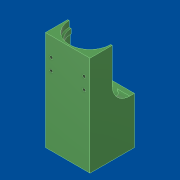
# Autodesk Inventor part: 402-gearbox-housing
Saved by Autodesk Inventor 2018 (Build 220112000, 112)
## iProperties
Created: 2020-06-11
Part Number: 402-gearbox-housing
Material: Generic
Document SubType Name: Modeling
Designer: Bunny320
Density: 1 g/cm^3
Appearance: Smooth - Dark Forest Green
Author: Bunny320
Autodesk Inventor part; units mm, degrees
ref_plane "YZ Plane" through (0, 0, 0) normal (1, 0, 0) x (0, 1, 0)
ref_plane "XZ Plane" through (0, 0, 0) normal (0, 1, 0) x (-1, 0, 0)
ref_plane "XY Plane" through (0, 0, 0) normal (0, 0, 1) x (1, 0, 0)
sketch "Sketch1" plane through (0, 0, 0) normal (0, 0, 1) x (1, 0, 0)
  line L0 (-19, -19) -> (19, -19)
  line L1 (19, -19) -> (19, 19)
  line L2 (19, 19) -> (-19, 19)
  line L3 (-19, 19) -> (-19, -19)
  line L4 (-19, -19) -> (19, 19) construction
  line L5 (19, -19) -> (-19, 19) construction
  point P0 (0, 0)
  dimension "d0" = 38
  constraints: 12 end point, 2 midpoint, 2 parallel, 2 perpendicular, 1 horizontal
  measures "d0" distance of L1.end L2.end
extrude "Extrusion1" add sketch "Sketch1" along normal blind 85
sketch "Sketch2" plane through (0, 0, 0) normal (0, 0, -1) x (-1, 0, 0)
  circle A0 centre (0, 0) radius 16.1
  dimension "d3" = 32.2
  constraints: 1 centre point, 1 coincident
  measures "d3" diameter of A0
extrude "Extrusion2" cut sketch "Sketch2" against normal blind 32
sketch "Sketch3" plane through (0, 0, 85) normal (0, 0, 1) x (1, 0, 0)
  circle A0 centre (0, 0) radius 17
  dimension "d6" = 34
  constraints: 1 centre point, 1 coincident
  measures "d6" diameter of A0
extrude "Extrusion3" cut sketch "Sketch3" against normal blind 45
sketch "Sketch4" plane through (0, 0, 40) normal (0, 0, 1) x (1, 0, 0)
  circle A0 centre (0, 0) radius 10
  dimension "d9" = 20
  constraints: 1 centre point, 1 coincident
  measures "d9" diameter of A0
extrude "Extrusion4" cut sketch "Sketch4" against normal through all
sketch "Sketch5" plane through (0, 0, 40) normal (0, 0, 1) x (1, 0, 0)
  point P0 (0, 0)
  point P1 (0, 13)
  dimension "d12" = 13
  constraints: 1 vertical alignment
  measures "d12" distance of point (0, 0) point (0, 13)
hole "Hole1" at (0, 13, 40) direction (0, 0, -1) diameter 3.4 end through all countersink diameter 7.5 countersink angle 90 clearance for "Countersunk Flat Head Hex Socket Screw DIN EN ISO 10642" size "M3" standard "DIN"
pattern_circular "Circular Pattern1" count 4 over 360 about axis through (0, 0, -10) along (0, 0, 1) of "Hole1"
sketch "Sketch7" plane through (0, 0, 0) normal (0, 1, 0) x (-1, 0, 0)
  line L0 (17, 55) -> (11, 55)
  line L1 (11, 55) -> (11, 63)
  line L2 (11, 63) -> (17, 63)
  line L3 (17, 85) -> (17, 40) projected
  line L4 (17, 63) -> (17, 55)
  line L5 (0, 87.7085) -> (0, 95.5721)
  line L6 (1.9638, 40) -> (9.8053, 40) projected
  line L7 (17, 77) -> (17, 64.9)
  line L8 (-17, 85) -> (17, 85) projected
  line L9 (17, 80) -> (16, 80)
  line L10 (16, 80) -> (16, 76)
  line L11 (16, 76) -> (17, 76)
  line L12 (17, 76) -> (17, 80)
  line L13 (17, 85) -> (17, 40) projected
  line L14 (-19, 0) -> (19, 0) projected
  line L15 (9.8053, 40) -> (16.75, 40) projected
  point P0 (0, 0)
  point P1 (0, 0)
  dimension "d27" = 22
  dimension "d39" = 5
  dimension "d40" = 9
  dimension "d41" = 32
  dimension "d90" = 8
  dimension "d92" = 15
  constraints: 21 end point, 4 perpendicular, 4 point on line, 2 collinear, 2 horizontal, 1 midpoint, 1 vertical
  measures "d27" diameter of L1 L5
  measures "d39" distance between parallel lines of L8 L9
  measures "d40" distance between parallel lines of L8 L11
  measures "d41" diameter of L10 L5
  measures "d90" distance between parallel lines of L2 L0
  measures "d92" distance between parallel lines of L15 L0
revolve "Revolution1" add sketch "Sketch7" angle 360 about axis through (0, 0, 87.7085) along (0, 0, 1)
sketch "Sketch8" plane through (0, 0, 85) normal (0, 0, 1) x (1, 0, 0)
  circle A0 centre (0, 0) radius 17.75
  dimension "d42" = 35.5
  constraints: 1 centre point, 1 coincident
  measures "d42" diameter of A0
extrude "Extrusion6" cut sketch "Sketch8" against normal up to surface (5 mm away)
sketch "Sketch10" plane through (-19, -19, 0) normal (0, -1, 0) x (1, 0, 0)
  line L0 (33, 70.95) -> (5, 70.95)
  line L1 (5, 70.95) -> (5, 65)
  line L2 (5, 65) -> (33, 65)
  line L3 (33, 65) -> (33, 70.95)
  line L4 (0, 0) -> (0, 85) projected
  line L5 (38, 0) -> (38, 85) projected
  point P0 (19, 0)
  dimension "d58" = 5
  dimension "d59" = 5
  constraints: 8 end point, 2 coincident, 2 parallel, 1 horizontal, 1 perpendicular
  measures "d58" distance between parallel lines of L4 L1
  measures "d59" distance between parallel lines of L5 L3
hole "Hole3" [suppressed]
sketch "Sketch11" plane through (0, 0, 85) normal (0, 0, 1) x (1, 0, 0)
  line L0 (19, 19) -> (-19, 19) projected
  line L1 (19, -19) -> (19, 19) projected
  line L2 (-19, 19) -> (19, 19)
  line L3 (19, 19) -> (19, 0)
  line L4 (19, 0) -> (-19, 0)
  line L5 (-19, 0) -> (-19, 19)
  point P0 (0, 0)
  constraints: 8 end point, 2 parallel, 1 horizontal, 1 midpoint, 1 perpendicular
extrude "Extrusion7" cut sketch "Sketch11" against normal up to surface (45 mm away)
sketch "Sketch12" plane through (-19, -19, 0) normal (0, -1, 0) x (1, 0, 0)
  line L0 (5, 59) -> (33, 59)
  line L1 (33, 59) -> (33, 69)
  line L2 (33, 69) -> (5, 69)
  line L3 (5, 69) -> (5, 59)
  line L4 (0, 0) -> (0, 85) projected
  line L5 (0, 0) -> (38, 0) projected
  line L6 (38, 0) -> (38, 85) projected
  point P0 (19, 0)
  dimension "d69" = 5
  dimension "d71" = 5
  dimension "d72" = 10
  dimension "d93" = 59
  constraints: 8 end point, 4 coincident, 2 parallel, 1 horizontal, 1 perpendicular
  measures "d69" distance between parallel lines of L4 L3
  measures "d71" distance between parallel lines of L6 L1
  measures "d72" distance of L0.end L1.end
  measures "d93" distance between parallel lines of L5 L0
hole "Hole4" at (-14, -19, 59) at (-14, -19, 69) at (14, -19, 59) at (14, -19, 69) direction (0, 1, 0) diameter 2.459 end through all thread size "M3x0.5" class "6H" standard "ISO Metric profile"
fillet "Fillet1" radius 15 2 edges at (-18, 0, 40) (18, 0, 40)
sketch "Sketch6" plane through (0, 0, 0) normal (0, 1, 0) x (-1, 0, 0)
  line L0 (-59.915, -50.2576) -> (49.2575, -50.2576)
  line L1 (49.2575, -50.2576) -> (49.2575, 450.4062)
  line L2 (49.2575, 450.4062) -> (-59.915, 450.4062)
  line L3 (-59.915, 450.4062) -> (-59.915, -50.2576)
  point P0 (0, 0)
  constraints: 8 end point, 2 parallel, 1 horizontal, 1 perpendicular
equation "\"d59\" = d58"
equation "\"d71\" = d69"
body "Solid1"
